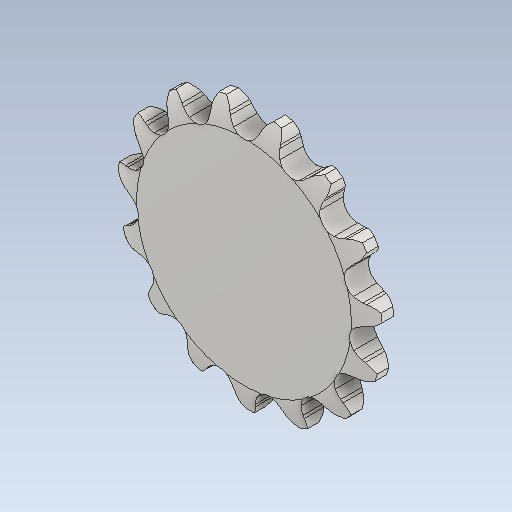
# Autodesk Inventor part: Roller Chain Sprocket2
Saved by Autodesk Inventor 2020 (Build 240168000, 168)
## iProperties
CustomPartVersion: 1
Created: 2021-01-09
Part Number: Roller Chain Sprocket2
Material: Steel
Document SubType Name: Modeling
Designer: lucky
Density: 7.85 g/cm^3
Appearance: Steel
Mass: 56.1792 g
Surface Area: 40.486 cm^2
Volume: 7.15659 cm^3
Author: lucky
Autodesk Inventor part; units mm, degrees
ref_plane "YZ Plane" through (0, 0, 0) normal (1, 0, 0) x (0, 1, 0)
ref_plane "XZ Plane" through (0, 0, 0) normal (0, 1, 0) x (-1, 0, 0)
sketch "Theoretical Tooth Profile" plane through (0, 0, 0) normal (0, 0, 1) x (1, 0, 0)
  circle A0 centre (0, 0) radius 22.9064 construction
  line L0 (0, 0) -> (0, 22.9064) construction
  line L1 (0, 0) -> (9.3169, 20.926) construction
  circle A1 centre (0, 0) radius 25.2633
  arc A2 (-2.0134, 21.2759) -> (2.0134, 21.2759) centre (0, 22.9064) ccw
  line L2 (0, 22.9064) -> (9.3169, 20.926) construction
  line L3 (0, 22.9064) -> (3.1583, 25.4639) construction
  line L4 (3.1583, 25.4639) -> (-2.886, 22.6796) construction
  arc A3 (4.4991, 24.8595) -> (3.1228, 23.1937) centre (6.9566, 21.4277) ccw
  arc A4 (-3.1228, 23.1937) -> (-4.4991, 24.8595) centre (-6.9566, 21.4277) ccw
  line L5 (-6.9566, 21.4277) -> (-3.1228, 23.1937) construction
  arc A5 (-2.886, 22.6796) -> (-2.0134, 21.2759) centre (3.1583, 25.4639) ccw
  line L6 (-2.886, 22.6796) -> (-3.1228, 23.1937)
  arc A6 (2.0134, 21.2759) -> (2.886, 22.6796) centre (-3.1583, 25.4639) ccw
  line L7 (3.1228, 23.1937) -> (2.886, 22.6796)
  line L8 (0, 0) -> (5.2525, 24.7112) construction
  point P0 (4.6584, 21.9162)
  dimension "d0" = 45.8127
  dimension "d2" = 24
  dimension "d3" = 2.5908
  dimension "d10" = 129
  dimension "d11" = 14.267
  dimension "d12" = 4.064
  dimension "d13" = 6.6548
  dimension "d14" = 7.112
  dimension "d23" = 2.8575
  constraints: 18 end point, 15 point on circle, 7 centre point, 3 coincident, 3 point on line, 3 symmetric about line, 3 tangent, 1 equal radius, 1 midpoint, 1 parallel, 1 vertical, 1 other
  measures "d0" diameter of A0
  measures "d2" angle of L1 L0
  measures "d3" radius of A2
  measures "d10" angle of L3 L0
  measures "d11" angle of L4 L3
  measures "d12" distance of L2.start L3.end
  measures "d13" distance of L3.end L4.end
  measures "d14" distance of A3.centre L0.end
  measures "d23" distance from line of L8.end L2
sketch "Tooth Profile" plane through (0, 0, 0) normal (0, 0, 1) x (1, 0, 0)
  arc A0 (-2.3848, 21.8941) -> (2.3848, 21.8941) centre (0, 22.9064) ccw
  arc A1 (4.3245, 24.8904) -> (2.3848, 21.8941) centre (11.9242, 17.8448) ccw
  arc A2 (-2.3848, 21.8941) -> (-4.3245, 24.8904) centre (-11.9242, 17.8448) ccw
  line L0 (0, 0) -> (0, 22.9064) construction
  line L1 (0, 22.9064) -> (2.3848, 21.8941) construction
  line L2 (0, 22.9064) -> (-2.3848, 21.8941) construction
  circle A3 centre (0, 0) radius 25.2633 projected
  dimension "d44" = 134
  dimension "d45" = 10.3632
  dimension "d46" = 2.5908
  constraints: 9 point on circle, 6 end point, 3 centre point, 2 tangent, 1 coincident, 1 equal radius, 1 vertical, 1 other
  measures "d44" angle of L2 L1
  measures "d45" radius of A1
  measures "d46" radius of A0
sketch "Section Profile" plane through (0, 0, 0) normal (1, 0, 0) x (0, 1, 0)
  line L0 (25.2633, 0) -> (-25.2633, 0) projected
  line L1 (16.8813, 2.2967) -> (-16.8813, 2.2967)
  line L2 (-16.8813, 2.2967) -> (-16.8813, -2.2967)
  line L3 (-16.8813, -2.2967) -> (16.8813, -2.2967)
  line L4 (16.8813, -2.2967) -> (16.8813, 2.2967)
  line L5 (16.8813, 2.2967) -> (25.2633, 2.2967) construction
  line L6 (25.2633, 2.2967) -> (25.2633, -2.2967) construction
  line L7 (25.2633, -2.2967) -> (16.8813, -2.2967) construction
  line L8 (16.8813, -2.2967) -> (16.8813, 2.2967)
  arc A0 (25.2633, 1.106) -> (20.4996, 2.2967) centre (20.4996, -7.8284) ccw
  arc A1 (20.4996, -2.2967) -> (25.2633, -1.106) centre (20.4996, 7.8284) ccw
  line L9 (20.4996, 2.2967) -> (0, 2.2967)
  line L10 (0, 2.2967) -> (0, -2.2967)
  line L11 (0, -2.2967) -> (20.4996, -2.2967)
  line L12 (0, 2.2967) -> (0, -2.2967)
  line L13 (25.2633, 1.106) -> (25.2633, -1.106)
  point P0 (0, 0)
  point P1 (0, 0)
  dimension "d30" = 4.5933
  dimension "d31" = 33.7626
  dimension "d32" = 4.5933
  dimension "d33" = 1.1906
  dimension "d34" = 10.1251
  dimension "d43" = 2.2967
  constraints: 26 end point, 7 midpoint, 5 perpendicular, 4 parallel, 4 point on circle, 3 point on line, 3 symmetric about line, 2 centre point, 2 horizontal, 2 tangent, 1 collinear, 1 other
  measures "d30" distance between parallel lines of L7 L5
  measures "d31" distance between parallel lines of L2 L4
  measures "d32" distance between parallel lines of L3 L1
  measures "d33" distance from line of L13.start L5
  measures "d34" radius of A0
  measures "d43" distance between parallel lines of L3 L0
revolve "Shroud" add sketch "Section Profile" angle 360 about axis through (0, 0, 2.2967) along (0, 0, -1) contours L10 L3 L2 L0 | L0 L2 L1 L10
revolve "Strand" add sketch "Section Profile" angle 360 about axis through (0, 0, 2.2967) along (0, 0, -1) contours L13 A1 L11 L4 L0 | L0 L4 L9 A0 L13 | L4 L3 L10 L0 | L0 L10 L1 L4
pattern_of_one "Strand Pattern"
extrude "Theoretical Tooth" cut sketch "Theoretical Tooth Profile" along normal through all both and the other way through all contours A3 L7 A6 A2 A5 L6 A4 A1 picked at (-0.5023, 22.59)
extrude "Tooth" [suppressed]
pattern_circular "Tooth Pattern" count 15 over 360 about axis through (0, 0, -10) along (0, 0, 1) of "Theoretical Tooth"
ref_plane "Timing Plane" through (0, 22.9064, 0) normal (1, 0, 0) x (0, 1, 0)
equation "\"d3\" = 0.5 * da_Dr + da_SC"
equation "\"d12\" = 0.8 * da_Dr"
equation "\"d13\" = 1.3 * da_Dr + da_SC"
equation "\"d14\" = 1.4 * da_Dr"
equation "\"d23\" = da_Ha"
equation "\"d44\" = da_Alfa"
equation "\"d45\" = da_Re"
equation "\"d46\" = da_Ri"
equation "\"d30\" = da_Bf"
equation "\"d31\" = da_Ds"
equation "\"d32\" = da_Bs"
equation "\"d33\" = da_Ba"
equation "\"d34\" = da_Rx"
equation "\"d40\" = da_pt"
equation "\"form_type\" = 0"
equation "\"da_p\" = 9.525"
equation "\"da_Dr\" = 5.08"
equation "\"da_SC\" = 0.0508"
equation "\"da_Ha\" = 2.8575"
equation "\"da_pt\" = 10.1346"
equation "\"da_Bf\" = 4.59334"
equation "\"da_Ba\" = 1.19063"
equation "\"da_Rx\" = 10.12508"
equation "\"da_Ra\" = 0.381"
equation "\"da_Bs\" = 4.59334"
equation "\"da_Ds\" = 33.7626"
equation "\"da_Re\" = 10.3632"
equation "\"da_Ri\" = 2.5908"
equation "\"da_Alfa\" = 134deg"
body "Solid1"
